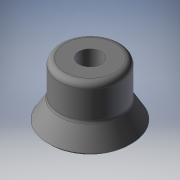
# Autodesk Inventor part: VP15AS
Saved by Autodesk Inventor 2019 (Build 230136000, 136)
## iProperties
Created: 2023-10-05
Part Number: VP15AS
Material: Generic
Catalog Web Link: www.cadenas.de
Description: VP_A-Pad Rubber only (Deep type)
Vendor: PISCO_JP
Document SubType Name: Modeling
Designer: psAdmin
Manufacturer: PISCO_JP
Mass: 0.670861 g
Surface Area: 7.64406 cm^2
Volume: 0.670861 cm^3
Density: 1 g/cm^3
Appearance: PSOLRGB-255-255-255
Category: PARTsolutions
Company: PISCO_JP
Title: VP15AS
Author: Cadenas PARTsolutions
Comments: Pad Rubber only (Deep type)
PSOL_IDENT_0: {$CADENAS_DATA/23d-libs/pisco_jp/vacuum_pad_series_r2/vacuum_pad_pad_and_holder_joint_assy/standard_
PSOL_IDENT_1: type/vp_a.prj},153 {VTYP=3D},{NB=VP15AS},{LINA=VP15AS},{NN=VP_A},{DATE=07.10.2020 11:38:13},{GEOMDAT
PSOL_IDENT_2: E=24.09.2019 08:02:00},{VERSION=},{LINEID=10},{WBVAR=PMS},{WBNUMERIC=}  {NB=VP15AS},{LINA=VP15AS},{K
PSOL_IDENT_3: T=DUMMY},{CNSORDERNO=VP15AS},{PD=15},{PCC=M4},{PTC=A},{PMS=S},{PMSX='N','N : Nitrile rubber','S','S
PSOL_IDENT_4: : Silicone rubber','U','U : Urethane rubber','F','F : Fluoro rubber','NE','NE : Conductive NBR(Low r
PSOL_IDENT_5: esistance type)','G','G : NBR Suited for the food sanitation act.','HN','HN : HNBR','EP','EP : EPDM'
PSOL_IDENT_6: },{COLOR=1.00,1.00,1.00,0.00}
NB: VP15AS
NN: VP_A
NT: Pad Rubber only (Deep type)
NBSYN: $CNSORDERNO.
LINA: VP15AS
CATALOG: NIHON PISCO CO., LTD
CNSORDERNO: VP15AS
PD: 15
PCC: M4
PTC: A
PMS: S : Silicone rubber
SUPPLIER: PISCO_JP
ARTICLENO: VP15AS
BOMINFO: VP15AS
CREATOR: CADENAS GmbH
Autodesk Inventor part; units mm, degrees
sketch "Sketch_1" plane through (0, 0, 0) normal (0, 0, 1) x (1, 0, 0)
  line L0 (0, 0) -> (0, 10)
  line L1 (2, 7) -> (3, 7)
  line L2 (3, 7) -> (3, 2.9235)
  arc A0 (7.0757, 0) -> (3, 2.9235) centre (0, -5.5618) ccw
  line L3 (7.0757, 0) -> (7.5, 0.4243)
  line L4 (7.5, 0.4243) -> (5.634, 3.6563)
  arc A1 (5.5, 4.1563) -> (5.634, 3.6563) centre (6.5, 4.1563) ccw
  line L5 (5.5, 4.1563) -> (5.5, 9)
  arc A2 (5.5, 9) -> (4.5, 10) centre (4.5, 9) ccw
  line L6 (4.5, 10) -> (2, 10)
  line L7 (2, 10) -> (2, 7)
  constraints: 16 end point, 6 point on circle, 3 centre point
revolve "Revolution1" add sketch "Sketch_1" angle 360 about axis through (0, 0, 0) along (0, -1, 0)
ref_plane "IP_dummy_XY" through (0, 0, 0) normal (0, 1, 0) x (1, 0, 0)
ref_plane "IP_dummy_YZ" through (0, 0, 0) normal (1, 0, 0) x (0, 0, -1)
ref_plane "IP_dummy_ZX" through (0, 0, 0) normal (0, 0, -1) x (0, 1, 0)
ref_plane "IP_screw_XY" through (0, 7, 0) normal (0, 1, 0) x (1, 0, 0)
ref_plane "IP_screw_YZ" through (0, 7, 0) normal (1, 0, 0) x (0, 0, -1)
ref_plane "IP_screw_ZX" through (0, 7, 0) normal (0, 0, -1) x (0, 1, 0)
body "Solid1"
